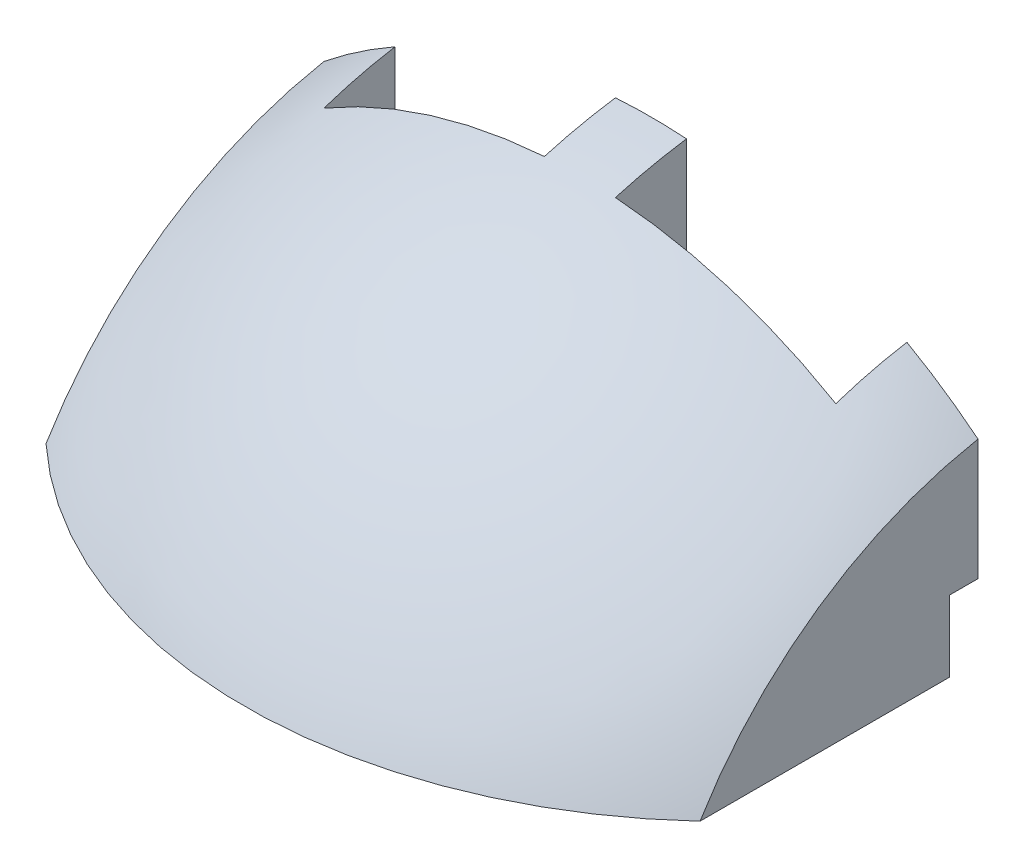
# Autodesk Inventor part: body back for main printing
Saved by Autodesk Inventor 2023 (Build 270158000, 158)
## iProperties
Created: 2022-10-08
Part Number: body back for main printing
Material: ABS プラスチック
Document SubType Name: Modeling
Designer: ellie
Density: 1.06 g/cm^3
Appearance: 積雪
Author: ellie
Autodesk Inventor part; units mm, degrees
sketch "スケッチ1" plane through (0, 0, 0) normal (0, 1, 0) x (-1, 0, 0)
  circle A0 centre (0, 0) radius 37
  line L0 (0, 0) -> (0, -37)
  line L1 (0, 0) -> (0, 37)
  dimension "d0" = 74
  constraints: 4 end point, 2 point on circle, 2 vertical, 1 centre point, 1 coincident
  measures "d0" diameter of A0
revolve "回転1" add sketch "スケッチ1" angle 180 about axis through (0, 0, 0) along (0, 0, 1) picked at (-2.7444, -24.3574) contours L1 L0 A0
sketch "スケッチ5" plane through (0, 0, 0) normal (0, -1, 0) x (1, 0, 0)
  line L0 (-20, -25) -> (20, -25)
  line L1 (20, -25) -> (20, -15)
  line L2 (20, -15) -> (-20, -15)
  line L3 (-20, -15) -> (-20, -25)
  line L4 (-20, -17) -> (-20, -15)
  line L5 (0, 27.75) -> (-17, 27.75)
  line L6 (-17, 27.75) -> (-17, 25.75)
  line L7 (-17, 25.75) -> (0, 25.75)
  line L8 (0, 25.75) -> (0, 27.75)
  line L9 (0, 22.75) -> (-20, 22.75)
  line L10 (-20, 22.75) -> (-20, 21.75)
  line L11 (-20, 21.75) -> (0, 21.75)
  line L12 (0, 21.75) -> (0, 22.75)
  line L13 (0, 15.75) -> (-21, 15.75)
  line L14 (-21, 15.75) -> (-21, 13.75)
  line L15 (-21, 13.75) -> (0, 13.75)
  line L16 (0, 13.75) -> (0, 15.75)
  line L17 (0, 7.75) -> (-23, 7.75)
  line L18 (-23, 7.75) -> (-23, 5.25)
  line L19 (-23, 5.25) -> (0, 5.25)
  line L20 (0, 5.25) -> (0, 7.75)
  circle A0 centre (0, 0) radius 37 projected
  circle A1 centre (0, 0) radius 37 projected
  line L21 (0, 37) -> (0, -37)
  line L22 (37, 0) -> (-37, 0)
  line L23 (-32.5, 5.25) -> (-23, 5.25)
  line L24 (-23, 5.25) -> (-23, -5.25)
  line L25 (-23, -5.25) -> (-32.5, -5.25)
  line L26 (-32.5, -5.25) -> (-32.5, 5.25)
  line L27 (-23, -8.0262) -> (-23, 5.25)
  line L28 (-27, 25.2982) -> (-27, -25.2982)
  line L29 (-15.5, 27.75) -> (-12, 27.75)
  line L30 (-12, 27.75) -> (-12, 35)
  line L31 (-12, 35) -> (-15.5, 35)
  line L32 (-15.5, 35) -> (-15.5, 27.75)
  line L33 (-15.5, 25.75) -> (0, 25.75)
  line L34 (0, 25.75) -> (0, 22.75)
  line L35 (0, 22.75) -> (-15.5, 22.75)
  line L36 (-15.5, 22.75) -> (-15.5, 25.75)
  line L37 (-19, 15.75) -> (0, 15.75)
  line L38 (0, 15.75) -> (0, 21.75)
  line L39 (0, 21.75) -> (-19, 21.75)
  line L40 (-19, 21.75) -> (-19, 15.75)
  line L41 (-19, 13.75) -> (0, 13.75)
  line L42 (0, 13.75) -> (0, 7.75)
  line L43 (0, 7.75) -> (-19, 7.75)
  line L44 (-19, 7.75) -> (-19, 13.75)
  line L45 (-23, 0) -> (-40.624, 0)
  line L46 (-23, 0) -> (-8.7712, 0)
  line L47 (-9.875, 5.25) -> (-23, 5.25)
  line L48 (-23, 5.25) -> (-23, -5.25)
  line L49 (-23, -5.25) -> (-9.875, -5.25)
  line L50 (-9.875, 5.25) -> (-23, -5.25) construction
  line L51 (-23, 5.25) -> (-9.875, -5.25) construction
  line L52 (-23, 7.25) -> (-33.5, 7.25)
  line L53 (-33.5, 7.25) -> (-33.5, -7.25)
  line L54 (-33.5, -7.25) -> (-23, -7.25)
  line L55 (-23, -7.25) -> (-23, 7.25)
  line L56 (-23, 7.25) -> (-33.5, -7.25) construction
  line L57 (-33.5, 7.25) -> (-23, -7.25) construction
  line L58 (-6.125, 5.25) -> (0, 5.25)
  line L59 (0, 5.25) -> (0, -5.25)
  line L60 (0, -5.25) -> (-6.125, -5.25)
  line L61 (-6.125, 5.25) -> (0, -5.25) construction
  line L62 (0, 5.25) -> (-6.125, -5.25) construction
  line L63 (-23, 5.25) -> (-27, 5.25)
  line L64 (-23, -5.25) -> (-27, -5.25)
  line L65 (-23, 7.25) -> (-27, 7.25)
  line L66 (-23, -7.25) -> (-27, -7.25)
  line L67 (26.3249, -26) -> (-26.3249, -26)
  line L68 (-6.125, 5.25) -> (-6.8, 5.25)
  line L69 (-6.2297, -5.25) -> (-6.125, -5.25)
  line L70 (-6.125, -5.25) -> (-6.125, 5.25)
  line L71 (-3, 7.75) -> (0, 7.75)
  line L72 (0, 22.75) -> (-4, 22.75)
  line L73 (-4, 21.75) -> (0, 21.75)
  line L74 (0, 21.75) -> (0, 22.75)
  line L75 (-6, 7.75) -> (-1, 7.75)
  line L76 (0, 5.25) -> (-6, 5.25)
  point P0 (0, -25)
  point P1 (0, -15)
  point P2 (0, 26.75)
  point P3 (0, 22.25)
  point P4 (0, 14.75)
  point P5 (0, 6.5)
  point P6 (-20, -20)
  point P7 (-27, -0.5262)
  point P8 (-27, -5.25)
  point P9 (-15.5, 24.25)
  point P10 (-15.5, 33.5969)
  point P11 (0, 27.75)
  point P12 (0, 37)
  point P13 (0, 25.75)
  point P14 (0, 13.75)
  point P15 (0, 15.75)
  point P16 (-27, 0)
  point P17 (-32.5, 0)
  point P18 (-23, 0)
  point P19 (-16.4375, 0)
  point P20 (-28.25, 0)
  point P21 (-3.0625, 0)
  point P22 (-27, 0.5)
  point P23 (-28, 0.4738)
  point P24 (-28, -11.5262)
  point P25 (-27, -11.5)
  point P26 (-23, -5.25)
  point P27 (-23, 5.25)
  point P28 (-23, -5.25)
  point P29 (0, 0)
  point P30 (-8, 6)
  point P31 (-26.3249, -26)
  point P32 (-8, -6)
  point P33 (0, 21.75)
  point P34 (0, 22.75)
  point P35 (-27, -7.25)
  point P36 (-27, 7.25)
  point P37 (-19, 10.75)
  dimension "d12" = 40
  dimension "d13" = 10
  dimension "d23" = 17
  dimension "d24" = 2
  dimension "d27" = 20
  dimension "d28" = 1
  dimension "d30" = 21
  dimension "d31" = 2
  dimension "d33" = 2.5
  dimension "d88" = 0
  dimension "d89" = 0
  dimension "d90" = 12
  dimension "d92" = 20
  dimension "d97" = 9.5
  dimension "d98" = 10.5
  dimension "d113" = 27
  dimension "d122" = 15.5
  dimension "d124" = 3
  dimension "d125" = 15.5
  dimension "d126" = 6
  dimension "d127" = 6
  dimension "d147" = 10.5
  dimension "d161" = 14.5
  dimension "d162" = 10.5
  dimension "d164" = 10.5
  dimension "d170" = 26
  dimension "d207" = 0
  dimension "d283" = 2
  dimension "d284" = 2
  dimension "d297" = 23
  constraints: 152 end point, 28 parallel, 20 horizontal, 16 midpoint, 16 perpendicular, 16 point on line, 10 collinear, 1 vertical, 20 other
  measures "d12" distance of L2.end L1.end
  measures "d13" distance of L1.end L0.end
  measures "d23" distance of L7.end L6.end
  measures "d24" distance of L6.end L5.end
  measures "d27" distance of L11.end L10.end
  measures "d28" distance of L10.end L9.end
  measures "d30" distance of L15.end L14.end
  measures "d31" distance of L14.end L13.end
  measures "d33" distance of L18.end L17.end
  measures "d89" distance from line of point (0, 0) L22
  measures "d90" distance from line of L0 point (0, -37)
  measures "d92" distance of the line from the sketch origin of L3
  measures "d97" distance of L24.end L25.end
  measures "d98" distance of L23.end L24.end
  measures "d113" distance of the line from the sketch origin of L28
  measures "d122" distance of the line from the sketch origin of L32
  measures "d124" distance of L33.end L34.end
  measures "d126" distance of L38.end L37.end
  measures "d127" distance of L41.end L42.end
  measures "d147" distance of L48.end L47.end
  measures "d161" distance between parallel lines of L54 L52
  measures "d162" distance between parallel lines of L48 L53
  measures "d164" distance between parallel lines of L60 L58
  measures "d170" distance between parallel lines of L67 L22
  measures "d207" distance between parallel lines of L47 L19
  measures "d283" distance from line of L14 point (-19, 10.75)
  measures "d284" distance between parallel lines of L14 L40
  measures "d297" distance between parallel lines of L27 L59
extrude "GNSボード" cut sketch "スケッチ5" against normal blind 16 contours L8 L7 L6 L5
extrude "GNSボード止めるよう" cut sketch "スケッチ5" against normal blind 15 contours L21 L5 L30 A0 | L30 L5 L32 A0 | L21 L9 L36 L7
extrude "アルミ板１" cut sketch "スケッチ5" against normal blind 20 contours L12 L11 L10 L9
extrude "メイン基板" cut sketch "スケッチ5" against normal blind 21 contours L15 L14 L13 L16
extrude "メイン止めるよう" cut sketch "スケッチ5" against normal blind 14.5 contours L17 L44 L15 L21 | L13 L40 L11 L21
extrude "アルミ板２" cut sketch "スケッチ5" against normal blind 20 contours L19 L18 L17 L20
extrude "電池ボックス入れ" cut sketch "スケッチ5" against normal blind 13 contours L3 L2 L21 L0 | L21 L2 L1 L0
extrude "side ut" cut sketch "スケッチ5" against normal blind 100 contours A0 L22 L53 L54 L28 | A0 L28 L52 L53 L22 | L54 L53 L22 L26 L25 L28 | L53 L52 L28 L23 L26 L22 | L25 L26 L22 L28 | L26 L23 L28 L22
extrude "motor case" add sketch "スケッチ5" against normal blind 7 contours L54 L53 L22 L26 L25 L28 | L28 L25 L27 L54 | L53 L52 L28 L23 L26 L22 | L28 L22 L24 L25 | L25 L26 L22 L28 | L22 L28 L23 L24 | L52 L18 L23 L28 | L26 L23 L28 L22
extrude "bottom cut" cut sketch "スケッチ5" against normal blind 90 contours L67 A0 L21 | L21 A0 L67
extrude "motor" [suppressed]
extrude "motor block" [suppressed]
sketch "スケッチ27" plane through (-33.5, 0, -7.25) normal (-1, 0, 0) x (0, 0, 1)
  line L0 (14.5, 0) -> (0, 0) projected
  circle A0 centre (7.25, 0) radius 3
  point P0 (7.25, 0)
  dimension "d198" = 6
  constraints: 1 centre point, 1 midpoint
  measures "d198" diameter of A0
extrude "押し出し36" cut sketch "スケッチ27" against normal blind 27
mirror "ミラー13" about plane through (0, 0, 0) normal (1, 0, 0) of "メイン止めるよう", "メイン基板", "アルミ板１", "GNSボード止めるよう", "GNSボード", "アルミ板２", "motor case", "押し出し36", "電池ボックス入れ", "side ut"
ref_plane "作業平面5" through (-17, 17.5, 25.75) normal (0, -1, 0) x (1, 0, 0)
ref_plane "作業平面6" through (20, 13, -15) normal (0, 0, -1) x (1, 0, 0)
sketch "スケッチ38" plane through (20, 13, -15) normal (0, 0, -1) x (1, 0, 0)
  line L0 (-40, 13) -> (0, 13) projected
  line L1 (-40, 13) -> (-40, 0) projected
  line L2 (-40, 0) -> (0, 0) projected
  line L3 (0, 13) -> (0, 0) projected
  line L4 (-38, 6) -> (-28, 6)
  line L5 (-28, 6) -> (-28, -3)
  line L6 (-28, -3) -> (-38, -3)
  line L7 (-38, -3) -> (-38, 6)
  point P0 (-20, 13)
  dimension "d235" = 3
  dimension "d236" = 9
  dimension "d237" = 10
  dimension "d238" = 2
  constraints: 8 end point, 2 parallel, 1 horizontal, 1 perpendicular
  measures "d235" distance between parallel lines of L6 L2
  measures "d236" distance between parallel lines of L6 L4
  measures "d237" distance between parallel lines of L7 L5
  measures "d238" distance between parallel lines of L1 L7
extrude "押し出し44" cut sketch "スケッチ38" against normal blind 18 contours L7 L4 L5 L2 | L2 L5 L6 L7
ref_plane "作業平面7" through (27, 35, 7.25) normal (0, -1, 0) x (1, 0, 0)
sketch "スケッチ41" plane through (-17, 0, 25.75) normal (0, -1, 0) x (1, 0, 0)
  line L0 (-16.5, -22.75) -> (10.5, -22.75) projected
  line L1 (-6, -20.5) -> (-6, -18) projected
  line L2 (-6, -18) -> (-2, -18) projected
  line L3 (-2, -18) -> (-2, -12) projected
  line L4 (-2, -12) -> (-4, -12) projected
  line L5 (-4, -12) -> (-4, -10) projected
  line L6 (-4, -10) -> (-2, -10) projected
  line L7 (-2, -10) -> (-2, -4) projected
  line L8 (-2, -4) -> (-3, -4) projected
  line L9 (-3, -4) -> (-3, -3) projected
  line L10 (-3, -3) -> (1.5, -3) projected
  line L11 (1.5, -3) -> (1.5, 0) projected
  line L12 (1.5, 0) -> (0, 0) projected
  line L13 (0, 0) -> (0, 2) projected
  line L14 (0, 2) -> (1.5, 2) projected
  line L15 (1.5, 2) -> (1.5, 7.8469) projected
  arc A0 (1.5, 7.8469) -> (-10, -0.4518) centre (17, -25.75) ccw projected
  line L16 (-10, -0.4518) -> (-10, -18.5) projected
  line L17 (-10, -18.5) -> (-16.5, -18.5) projected
  line L18 (-16.5, -18.5) -> (-16.5, -22.75) projected
  line L19 (-2, -18) -> (-2, -12) projected
  line L20 (-4, -10) -> (-4, -12) projected
  line L21 (0, 2) -> (0, 0) projected
  circle A1 centre (-4, 0) radius 2
  line L22 (50.5, -28.75) -> (23.5, -28.75) projected
  line L23 (23.5, -28.75) -> (23.5, -22.75) projected
  line L24 (23.5, -22.75) -> (50.5, -22.75) projected
  line L25 (50.5, -18.5) -> (50.5, -22.75) projected
  line L26 (44, -18.5) -> (50.5, -18.5) projected
  line L27 (44, -18.5) -> (44, -0.4518) projected
  arc A2 (44, -0.4518) -> (32.5, 7.8469) centre (17, -25.75) ccw projected
  line L28 (32.5, 7.8469) -> (32.5, 2) projected
  line L29 (32.5, 2) -> (34, 2) projected
  line L30 (34, 2) -> (34, 0) projected
  line L31 (34, 0) -> (32.5, 0) projected
  line L32 (32.5, 0) -> (32.5, -3) projected
  line L33 (32.5, -3) -> (37, -3) projected
  line L34 (37, -3) -> (37, -4) projected
  line L35 (37, -4) -> (36, -4) projected
  line L36 (36, -4) -> (36, -10) projected
  line L37 (36, -10) -> (38, -10) projected
  line L38 (38, -10) -> (38, -12) projected
  line L39 (38, -12) -> (36, -12) projected
  line L40 (36, -12) -> (36, -18) projected
  line L41 (36, -18) -> (40, -18) projected
  line L42 (40, -18) -> (40, -20.5) projected
  line L43 (40, -20.5) -> (-6, -20.5) projected
  line L44 (10.5, -22.75) -> (10.5, -28.75) projected
  line L45 (10.5, -28.75) -> (-16.5, -28.75) projected
  line L46 (-16.5, -28.75) -> (-16.5, -33) projected
  line L47 (-16.5, -33) -> (-10, -33) projected
  line L48 (-10, -33) -> (-10, -51.0482) projected
  arc A3 (-10, -51.0482) -> (-9.3249, -51.75) centre (17, -25.75) ccw projected
  line L49 (-9.3249, -51.75) -> (43.3249, -51.75) projected
  arc A4 (43.3249, -51.75) -> (44, -51.0482) centre (17, -25.75) ccw projected
  line L50 (44, -51.0482) -> (44, -33) projected
  line L51 (50.5, -33) -> (44, -33) projected
  line L52 (50.5, -28.75) -> (50.5, -33) projected
  dimension "d252" = 4
  dimension "d253" = 4
  dimension "d254" = 3
  constraints: 1 centre point
  measures "d252" diameter of A1
  measures "d253" distance from line of A1.centre L13
  measures "d254" distance from line of A1.centre L10
extrude "押し出し46" cut sketch "スケッチ41" against normal blind 10 contours A1
mirror "ミラー15" about plane through (0, 0, 0) normal (1, 0, 0) of "押し出し46"
sketch "スケッチ42" plane through (-33.5, 0, -7.25) normal (0, -1, 0) x (1, 0, 0)
  circle A0 centre (10, -8) radius 2
  line L0 (13.5, -17.75) -> (13.5, -7.75) projected
  line L1 (10, 2) -> (1, 2) projected
  point P0 (33.5, 7.25)
  dimension "d257" = 3.5
  dimension "d258" = 4
  dimension "d259" = 10
  constraints: 1 centre point
  measures "d257" distance from line of A0.centre L0
  measures "d258" diameter of A0
  measures "d259" distance from line of A0.centre L1
extrude "押し出し47" cut sketch "スケッチ42" against normal blind 10
mirror "ミラー16" about plane through (0, 0, 0) normal (1, 0, 0) of "押し出し47"
ref_plane "作業平面8" through (-17, 15, 25.75) normal (0, -1, 0) x (1, 0, 0)
sketch "スケッチ45" plane through (-17, 15, 25.75) normal (0, -1, 0) x (1, 0, 0)
  circle A0 centre (-4, 0) radius 2 projected
  line L0 (-16.5, -22.75) -> (10.5, -22.75) projected
  line L1 (-6, -20.5) -> (-6, -18) projected
  line L2 (-6, -18) -> (-2, -18) projected
  line L3 (-2, -18) -> (-2, -12) projected
  line L4 (-2, -12) -> (-4, -12) projected
  line L5 (-4, -12) -> (-4, -10) projected
  line L6 (-4, -10) -> (-2, -10) projected
  line L7 (-2, -10) -> (-2, -4) projected
  line L8 (-2, -4) -> (-3, -4) projected
  line L9 (-3, -4) -> (-3, -3) projected
  line L10 (-3, -3) -> (1.5, -3) projected
  line L11 (1.5, -3) -> (1.5, 0) projected
  line L12 (1.5, 0) -> (0, 0) projected
  line L13 (0, 0) -> (0, 2) projected
  line L14 (0, 2) -> (1.5, 2) projected
  line L15 (1.5, 2) -> (1.5, 7.8469) projected
  arc A1 (1.5, 7.8469) -> (-10, -0.4518) centre (17, -25.75) ccw projected
  line L16 (-10, -0.4518) -> (-10, -18.5) projected
  line L17 (-10, -18.5) -> (-16.5, -18.5) projected
  line L18 (-16.5, -18.5) -> (-16.5, -22.75) projected
  arc A2 (32.5, 4.3124) -> (1.5, 4.3124) centre (17, -25.75) ccw projected
  line L19 (1.5, 2) -> (1.5, 4.3124) projected
  line L20 (32.5, 2) -> (1.5, 2) projected
  line L21 (32.5, 2) -> (32.5, 4.3124) projected
  circle A3 centre (38, 0) radius 2 projected
  circle A4 centre (38, 0) radius 2 projected
  line L22 (23.5, -22.75) -> (50.5, -22.75) projected
  line L23 (50.5, -18.5) -> (50.5, -22.75) projected
  line L24 (44, -18.5) -> (50.5, -18.5) projected
  line L25 (44, -18.5) -> (44, -0.4518) projected
  arc A5 (44, -0.4518) -> (32.5, 7.8469) centre (17, -25.75) ccw projected
  line L26 (32.5, 7.8469) -> (32.5, 2) projected
  line L27 (32.5, 2) -> (34, 2) projected
  line L28 (34, 2) -> (34, 0) projected
  line L29 (34, 0) -> (32.5, 0) projected
  line L30 (32.5, 0) -> (32.5, -3) projected
  line L31 (32.5, -3) -> (37, -3) projected
  line L32 (37, -3) -> (37, -4) projected
  line L33 (37, -4) -> (36, -4) projected
  line L34 (36, -4) -> (36, -10) projected
  line L35 (36, -10) -> (38, -10) projected
  line L36 (38, -10) -> (38, -12) projected
  line L37 (38, -12) -> (36, -12) projected
  line L38 (36, -12) -> (36, -18) projected
  line L39 (36, -18) -> (40, -18) projected
  line L40 (40, -18) -> (40, -20.5) projected
  circle A6 centre (-4, 0) radius 2 projected
  line L41 (1.5, 0) -> (32.5, 0) projected
  line L42 (32.5, -3) -> (1.5, -3) projected
  line L43 (32.5, -3) -> (32.5, 0) projected
  line L44 (1.5, 0) -> (32.5, 0) projected
  line L45 (1.5, -3) -> (1.5, 0) projected
  line L46 (34, 0) -> (0, 0) projected
  line L47 (34, 0) -> (34, 2) projected
  line L48 (34, 2) -> (0, 2) projected
  line L49 (0, 0) -> (0, 2) projected
  line L50 (36, -10) -> (-2, -10) projected
  line L51 (36, -10) -> (36, -4) projected
  line L52 (-2, -4) -> (36, -4) projected
  line L53 (-2, -10) -> (-2, -4) projected
  line L54 (38, -12) -> (-4, -12) projected
  line L55 (38, -12) -> (38, -10) projected
  line L56 (38, -10) -> (-4, -10) projected
  line L57 (-4, -12) -> (-4, -10) projected
  line L58 (36, -18) -> (-2, -18) projected
  line L59 (36, -18) -> (36, -12) projected
  line L60 (-2, -12) -> (36, -12) projected
  line L61 (-2, -18) -> (-2, -12) projected
  line L62 (40, -20.5) -> (-6, -20.5) projected
  line L63 (40, -20.5) -> (40, -18) projected
  line L64 (40, -18) -> (-6, -18) projected
  line L65 (-6, -20.5) -> (-6, -18) projected
  circle A7 centre (40.5, -41) radius 2 projected
  circle A8 centre (-6.5, -41) radius 2 projected
  line L66 (50.5, -28.75) -> (23.5, -28.75) projected
  line L67 (40, -20.5) -> (-6, -20.5) projected
  line L68 (10.5, -28.75) -> (-16.5, -28.75) projected
  line L69 (-6, -20.5) -> (-6, -18) projected
  line L70 (-16.5, -28.75) -> (-16.5, -33) projected
  line L71 (-16.5, -33) -> (-10, -33) projected
  line L72 (-10, -33) -> (-10, -51.0482) projected
  arc A9 (-10, -51.0482) -> (-9.3249, -51.75) centre (17, -25.75) ccw projected
  line L73 (-9.3249, -51.75) -> (43.3249, -51.75) projected
  arc A10 (43.3249, -51.75) -> (44, -51.0482) centre (17, -25.75) ccw projected
  line L74 (44, -51.0482) -> (44, -33) projected
  line L75 (50.5, -33) -> (44, -33) projected
  line L76 (50.5, -28.75) -> (50.5, -33) projected
  line L77 (40, -18) -> (40, -20.5) projected
  line L78 (-3, -40.75) -> (37, -40.75) projected
  line L79 (37, -40.75) -> (37, -50.75) projected
  line L80 (37, -50.75) -> (-3, -50.75) projected
  line L81 (-3, -50.75) -> (-3, -40.75) projected
  line L82 (-6, -18) -> (40, -18)
  line L83 (40, -18) -> (40, 8.0731)
  line L84 (40, 8.0731) -> (-6, 8.0731)
  line L85 (-6, 8.0731) -> (-6, -18)
  arc A11 (32.5, 4.3124) -> (1.5, 4.3124) centre (17, -25.75) ccw projected
  line L86 (32.5, 4.3124) -> (32.5, 7.8469) projected
  arc A12 (44, -0.4518) -> (32.5, 7.8469) centre (17, -25.75) ccw projected
  line L87 (44, -0.4518) -> (44, -51.0482) projected
  arc A13 (43.3249, -51.75) -> (44, -51.0482) centre (17, -25.75) ccw projected
  line L88 (43.3249, -51.75) -> (-9.3249, -51.75) projected
  arc A14 (-10, -51.0482) -> (-9.3249, -51.75) centre (17, -25.75) ccw projected
  line L89 (-10, -51.0482) -> (-10, -0.4518) projected
  arc A15 (1.5, 7.8469) -> (-10, -0.4518) centre (17, -25.75) ccw projected
  line L90 (1.5, 7.8469) -> (1.5, 4.3124) projected
  line L91 (9, -32) -> (9, -20) projected
  line L92 (-6, -20) -> (9, -20) projected
  line L93 (-6, -21) -> (-6, -20) projected
  line L94 (-15, -21) -> (-6, -21) projected
  line L95 (-15, -31) -> (-15, -21) projected
  line L96 (-6, -31) -> (-15, -31) projected
  line L97 (-6, -32) -> (-6, -31) projected
  line L98 (9, -32) -> (-6, -32) projected
  line L99 (50.5, -28.75) -> (23.5, -28.75) projected
  line L100 (50.5, -22.75) -> (50.5, -28.75) projected
  line L101 (23.5, -22.75) -> (50.5, -22.75) projected
  line L102 (-16.5, -22.75) -> (10.5, -22.75) projected
  line L103 (-16.5, -28.75) -> (-16.5, -22.75) projected
  line L104 (10.5, -28.75) -> (-16.5, -28.75) projected
  line L105 (10.5, -28.75) -> (10.5, -22.75) projected
  line L106 (23.5, -28.75) -> (23.5, -22.75) projected
  line L107 (50.5, -28.75) -> (23.5, -28.75) projected
  line L108 (23.5, -28.75) -> (23.5, -22.75) projected
  line L109 (40, -20.5) -> (-6, -20.5) projected
  line L110 (-6, -20.5) -> (-6, -18) projected
  line L111 (-6, -18) -> (-2, -18) projected
  line L112 (-2, -18) -> (-2, -12) projected
  line L113 (-2, -12) -> (-4, -12) projected
  line L114 (-4, -12) -> (-4, -10) projected
  line L115 (-4, -10) -> (-2, -10) projected
  line L116 (-2, -10) -> (-2, -4) projected
  line L117 (-2, -4) -> (-3, -4) projected
  line L118 (-3, -4) -> (-3, -3) projected
  line L119 (-3, -3) -> (1.5, -3) projected
  line L120 (1.5, -3) -> (1.5, 0) projected
  line L121 (1.5, 0) -> (0, 0) projected
  line L122 (0, 0) -> (0, 2) projected
  line L123 (0, 2) -> (1.5, 2) projected
  line L124 (1.5, 2) -> (1.5, 7.8469) projected
  arc A16 (1.5, 7.8469) -> (-10, -0.4518) centre (17, -25.75) ccw projected
  line L125 (-10, -0.4518) -> (-10, -18.5) projected
  line L126 (-10, -18.5) -> (-16.5, -18.5) projected
  line L127 (-16.5, -18.5) -> (-16.5, -22.75) projected
  line L128 (-16.5, -22.75) -> (10.5, -22.75) projected
  line L129 (10.5, -22.75) -> (10.5, -28.75) projected
  line L130 (10.5, -28.75) -> (-16.5, -28.75) projected
  line L131 (-16.5, -28.75) -> (-16.5, -33) projected
  line L132 (-16.5, -33) -> (-10, -33) projected
  line L133 (-10, -33) -> (-10, -51.0482) projected
  arc A17 (-10, -51.0482) -> (-9.3249, -51.75) centre (17, -25.75) ccw projected
  line L134 (-9.3249, -51.75) -> (43.3249, -51.75) projected
  arc A18 (43.3249, -51.75) -> (44, -51.0482) centre (17, -25.75) ccw projected
  line L135 (44, -51.0482) -> (44, -33) projected
  line L136 (50.5, -33) -> (44, -33) projected
  line L137 (50.5, -28.75) -> (50.5, -33) projected
  line L138 (50.5, -28.75) -> (23.5, -28.75) projected
  line L139 (23.5, -28.75) -> (23.5, -22.75) projected
  line L140 (23.5, -22.75) -> (50.5, -22.75) projected
  line L141 (50.5, -18.5) -> (50.5, -22.75) projected
  line L142 (44, -18.5) -> (50.5, -18.5) projected
  line L143 (44, -18.5) -> (44, -0.4518) projected
  arc A19 (44, -0.4518) -> (32.5, 7.8469) centre (17, -25.75) ccw projected
  line L144 (32.5, 7.8469) -> (32.5, 2) projected
  line L145 (32.5, 2) -> (34, 2) projected
  line L146 (34, 2) -> (34, 0) projected
  line L147 (34, 0) -> (32.5, 0) projected
  line L148 (32.5, 0) -> (32.5, -3) projected
  line L149 (32.5, -3) -> (37, -3) projected
  line L150 (37, -3) -> (37, -4) projected
  line L151 (37, -4) -> (36, -4) projected
  line L152 (36, -4) -> (36, -10) projected
  line L153 (36, -10) -> (38, -10) projected
  line L154 (38, -10) -> (38, -12) projected
  line L155 (38, -12) -> (36, -12) projected
  line L156 (36, -12) -> (36, -18) projected
  line L157 (36, -18) -> (40, -18) projected
  line L158 (40, -18) -> (40, -20.5) projected
  line L159 (40, -20.5) -> (-6, -20.5) projected
  line L160 (10.5, -22.75) -> (10.5, -28.75) projected
  line L161 (10.5, -28.75) -> (-16.5, -28.75) projected
  line L162 (-16.5, -28.75) -> (-16.5, -33) projected
  line L163 (-16.5, -33) -> (-10, -33) projected
  line L164 (-10, -33) -> (-10, -51.0482) projected
  arc A20 (-10, -51.0482) -> (-9.3249, -51.75) centre (17, -25.75) ccw projected
  line L165 (-9.3249, -51.75) -> (43.3249, -51.75) projected
  arc A21 (43.3249, -51.75) -> (44, -51.0482) centre (17, -25.75) ccw projected
  line L166 (44, -51.0482) -> (44, -33) projected
  line L167 (50.5, -33) -> (44, -33) projected
  line L168 (50.5, -28.75) -> (50.5, -33) projected
  line L169 (23.5, -28.75) -> (23.5, -22.75) projected
  line L170 (23.5, -22.75) -> (50.5, -22.75) projected
  line L171 (50.5, -18.5) -> (50.5, -22.75) projected
  line L172 (44, -18.5) -> (50.5, -18.5) projected
  line L173 (44, -18.5) -> (44, -0.4518) projected
  arc A22 (44, -0.4518) -> (32.5, 7.8469) centre (17, -25.75) ccw projected
  line L174 (32.5, 7.8469) -> (32.5, 2) projected
  line L175 (32.5, 2) -> (34, 2) projected
  line L176 (34, 2) -> (34, 0) projected
  line L177 (34, 0) -> (32.5, 0) projected
  line L178 (32.5, 0) -> (32.5, -3) projected
  line L179 (32.5, -3) -> (37, -3) projected
  line L180 (37, -3) -> (37, -4) projected
  line L181 (37, -4) -> (36, -4) projected
  line L182 (36, -4) -> (36, -10) projected
  line L183 (36, -10) -> (38, -10) projected
  line L184 (38, -10) -> (38, -12) projected
  line L185 (38, -12) -> (36, -12) projected
  line L186 (36, -12) -> (36, -18) projected
  line L187 (36, -18) -> (40, -18) projected
  line L188 (-6, -18) -> (-2, -18) projected
  line L189 (-2, -18) -> (-2, -12) projected
  line L190 (-2, -12) -> (-4, -12) projected
  line L191 (-4, -12) -> (-4, -10) projected
  line L192 (-4, -10) -> (-2, -10) projected
  line L193 (-2, -10) -> (-2, -4) projected
  line L194 (-2, -4) -> (-3, -4) projected
  line L195 (-3, -4) -> (-3, -3) projected
  line L196 (-3, -3) -> (1.5, -3) projected
  line L197 (1.5, -3) -> (1.5, 0) projected
  line L198 (1.5, 0) -> (0, 0) projected
  line L199 (0, 0) -> (0, 2) projected
  line L200 (0, 2) -> (1.5, 2) projected
  line L201 (1.5, 2) -> (1.5, 7.8469) projected
  arc A23 (1.5, 7.8469) -> (-10, -0.4518) centre (17, -25.75) ccw projected
  line L202 (-10, -0.4518) -> (-10, -18.5) projected
  line L203 (-10, -18.5) -> (-16.5, -18.5) projected
  line L204 (-16.5, -18.5) -> (-16.5, -22.75) projected
  line L205 (-16.5, -22.75) -> (10.5, -22.75) projected
  line L206 (10.5, -22.75) -> (10.5, -28.75) projected
  point P0 (-10, -33)
  point P1 (44, -33)
  point P2 (44, -18.5)
  point P3 (40, 3.2328)
  point P4 (40, -18)
  point P5 (-6, -20.5)
  point P6 (-6, -18)
  point P7 (-6, 3.2328)
  point P8 (-10, -33)
  point P9 (44, -33)
  point P10 (44, -18.5)
  point P11 (-10, -18.5)
  point P12 (44, -22.75)
  point P13 (-10, -22.75)
  point P14 (-10, -18.5)
  point P15 (44, -28.75)
  point P16 (-10, -28.75)
  point P17 (32.5, 4.3124)
  point P18 (1.5, 4.3124)
  point P19 (1.5, 4.3124)
  point P20 (32.5, 4.3124)
  point P21 (-10, -22.75)
  point P22 (-10, -28.75)
  point P23 (32.5, 4.3124)
  point P24 (1.5, 4.3124)
  point P25 (44, -22.75)
  point P26 (44, -28.75)
  point P27 (-10, -18.5)
  point P28 (50.5, -28.75)
  point P29 (44, -33)
  point P30 (1.5, 4.3124)
  point P31 (32.5, 4.3124)
  point P32 (50.5, -28.75)
  point P33 (44, -28.75)
  point P34 (44, -22.75)
  point P35 (32.5, 4.3124)
  point P36 (1.5, 4.3124)
  point P37 (44, -33)
  point P38 (-10, -22.75)
  point P39 (-10, -28.75)
  point P40 (1.5, 4.3124)
  point P41 (32.5, 4.3124)
  point P42 (-16.5, -28.75)
  point P43 (-16.5, -28.75)
  constraints: 8 end point, 3 collinear, 2 parallel, 1 horizontal, 1 perpendicular, 1 tangent
extrude "side and front cut" cut sketch "スケッチ45" along normal mid plane 100 contours L85 L1 L93 L94 L89 L16 A1 | L89 L94 L95 L0 L18 L17 | L62 L91 L0 L89 L94 L93 | L89 L0 L95 L94 | L62 L40 L83 A5 L25 L87 L22 L106 L66 L74 A10 L73 A9 L72 L89 L96 L97 L98 L91 L68 L105 L0 | L0 L95 L68 L103 | L89 L68 L95 L0 | L0 L91 L68 L89 | L0 L105 L68 L91 | L68 L95 L96 L89 L71 L70 | L89 L96 L95 L68 | L68 L91 L98 L97 L96 L89 | L24 L23 L22 L87 | L87 L66 L106 L22 | L22 L100 L66 L87 | L66 L76 L75 L87 | A7 | A8 | L78 L79 L80 L81
sketch "スケッチ46" plane through (-17, 15, 25.75) normal (0, -1, 0) x (1, 0, 0)
  line L0 (-6, 0) -> (-6, -18) projected
  line L1 (-6, -18) -> (-2, -18) projected
  line L2 (-2, -18) -> (-2, -12) projected
  line L3 (-2, -12) -> (-4, -12) projected
  line L4 (-4, -12) -> (-4, -10) projected
  line L5 (-4, -10) -> (-2, -10) projected
  line L6 (-2, -10) -> (-2, -4) projected
  line L7 (-2, -4) -> (-3, -4) projected
  line L8 (-3, -4) -> (-3, -3) projected
  line L9 (-3, -3) -> (1.5, -3) projected
  line L10 (1.5, -3) -> (1.5, 0) projected
  line L11 (1.5, 0) -> (0, 0) projected
  line L12 (0, 0) -> (0, 2) projected
  line L13 (0, 2) -> (1.5, 2) projected
  line L14 (1.5, 2) -> (1.5, 7.8469) projected
  arc A0 (1.5, 7.8469) -> (-6, 3.2328) centre (17, -25.75) ccw projected
  line L15 (-6, 3.2328) -> (-6, 0) projected
  circle A1 centre (-4, 0) radius 2 projected
  circle A2 centre (-4, 0) radius 2 projected
  line L16 (40, -18) -> (40, 0) projected
  circle A3 centre (38, 0) radius 2 projected
  line L17 (40, 0) -> (40, 3.2328) projected
  arc A4 (40, 3.2328) -> (32.5, 7.8469) centre (17, -25.75) ccw projected
  line L18 (32.5, 7.8469) -> (32.5, 2) projected
  line L19 (32.5, 2) -> (34, 2) projected
  line L20 (34, 2) -> (34, 0) projected
  line L21 (34, 0) -> (32.5, 0) projected
  line L22 (32.5, 0) -> (32.5, -3) projected
  line L23 (32.5, -3) -> (37, -3) projected
  line L24 (37, -3) -> (37, -4) projected
  line L25 (37, -4) -> (36, -4) projected
  line L26 (36, -4) -> (36, -10) projected
  line L27 (36, -10) -> (38, -10) projected
  line L28 (38, -10) -> (38, -12) projected
  line L29 (38, -12) -> (36, -12) projected
  line L30 (36, -12) -> (36, -18) projected
  line L31 (36, -18) -> (40, -18) projected
  arc A5 (32.5, 4.3124) -> (1.5, 4.3124) centre (17, -25.75) ccw projected
  line L32 (1.5, 2) -> (1.5, 4.3124) projected
  line L33 (32.5, 2) -> (1.5, 2) projected
  line L34 (32.5, 2) -> (32.5, 4.3124) projected
  line L35 (34, 0) -> (0, 0) projected
  line L36 (34, 0) -> (34, 2) projected
  line L37 (34, 2) -> (0, 2) projected
  line L38 (0, 0) -> (0, 2) projected
  line L39 (32.5, -3) -> (1.5, -3) projected
  line L40 (32.5, -3) -> (32.5, 0) projected
  line L41 (1.5, 0) -> (32.5, 0) projected
  line L42 (1.5, -3) -> (1.5, 0) projected
  line L43 (36, -10) -> (-2, -10) projected
  line L44 (36, -10) -> (36, -4) projected
  line L45 (-2, -4) -> (36, -4) projected
  line L46 (-2, -10) -> (-2, -4) projected
  line L47 (36, -18) -> (-2, -18) projected
  line L48 (36, -18) -> (36, -12) projected
  line L49 (-2, -12) -> (36, -12) projected
  line L50 (-2, -18) -> (-2, -12) projected
  point P0 (1.5, 4.3124)
  point P1 (-2, -18)
  point P2 (36, -18)
  constraints: 3 horizontal alignment
extrude "front cut 2" cut sketch "スケッチ46" along normal blind 100 contours L15 A0 L14 L13 L12 L11 L10 L9 L8 L7 L6 L5 L4 L3 L2 L1 L0 | A1 | L2 L49 L30 L47 | L3 L4 L5 L43 L27 L28 L29 L49 | A3 | L30 L29 L28 L27 L26 L25 L24 L23 L22 L21 L20 L19 L18 A4 L17 L16 L31 | A5 L18 L33 L14 | L33 L19 L20 L21 L35 L11 L12 L13 | L6 L45 L26 L43 | L7 L8 L9 L39 L23 L24 L25 L45 | L35 L22 L39 L10
sketch "スケッチ48" plane through (0, 0, 5.25) normal (0, 0, -1) x (-1, 0, 0)
  line L0 (-23, 20) -> (23, 20) projected
  line L1 (23, 28.5033) -> (23, 20) projected
  arc A0 (23, 28.5033) -> (-23, 28.5033) centre (0, 0) ccw projected
  line L2 (-23, 28.5033) -> (-23, 20) projected
  line L3 (-23, 15) -> (23, 15) projected
  line L4 (-23, 15) -> (-23, 20) projected
  line L5 (23, 15) -> (23, 20) projected
  line L6 (-23, 40) -> (-18, 40)
  line L7 (-18, 40) -> (-18, 15)
  line L8 (-18, 15) -> (-23, 15)
  line L9 (-23, 15) -> (-23, 40)
  line L10 (18, 40) -> (23, 40)
  line L11 (23, 40) -> (23, 15)
  line L12 (23, 15) -> (18, 15)
  line L13 (18, 15) -> (18, 40)
  line L14 (-2.5, 36.6256) -> (2.5, 36.6256)
  line L15 (2.5, 36.6256) -> (2.5, 20)
  line L16 (2.5, 20) -> (-2.5, 20)
  line L17 (-2.5, 20) -> (-2.5, 36.6256)
  line L18 (0, 0) -> (0, 36.6256)
  point P0 (18, 20)
  point P1 (18, 31.8973)
  point P2 (-18, 31.8973)
  point P3 (-18, 20)
  point P4 (2.5, 36.5402)
  point P5 (2.5, 20)
  point P6 (-2.5, 36.5402)
  dimension "d274" = 25
  dimension "d275" = 5
  dimension "d276" = 25
  dimension "d277" = 5
  dimension "d280" = 5
  dimension "d282" = 2.5
  constraints: 26 end point, 6 parallel, 5 collinear, 3 horizontal, 3 perpendicular, 1 midpoint, 1 point on circle, 1 tangent
  measures "d274" distance between parallel lines of L3 L6
  measures "d275" distance between parallel lines of L9 L7
  measures "d276" distance between parallel lines of L3 L10
  measures "d277" distance between parallel lines of L13 L11
  measures "d280" distance between parallel lines of L17 L15
  measures "d282" distance between parallel lines of L17 L18
extrude "lock cut" cut sketch "スケッチ48" against normal blind 3 contours L7 A0 L17 L0 | L15 A0 L13 L0
sketch "スケッチ49" plane through (23, 15, 7.75) normal (0, 0, -1) x (-1, 0, 0)
  line L0 (46, 0) -> (0, 0) projected
  line L1 (46, -15) -> (46, 5) projected
  line L2 (0, 0) -> (46, 0)
  line L3 (46, 0) -> (46, 5)
  line L4 (46, 5) -> (0, 5)
  line L5 (0, 5) -> (0, 0)
  point P0 (23, -15)
  point P1 (38.5, 0)
  point P2 (7.5, 0)
  constraints: 8 end point, 2 parallel, 1 horizontal, 1 perpendicular
extrude "押し出し52" cut sketch "スケッチ49" against normal up to surface (0.5 mm away)
sketch "スケッチ50" plane through (0, 0, 5.25) normal (0, 0, -1) x (-1, 0, 0)
  point P0 (0, 0)
sketch "スケッチ51" plane through (0, 0, 8.25) normal (0, 0, -1) x (-1, 0, 0)
  line L0 (-23, 15) -> (-23, 28.5033) projected
  line L1 (18, 20) -> (23, 20) projected
  line L2 (-23, 15) -> (23, 15)
  line L3 (23, 15) -> (23, 20)
  line L4 (23, 20) -> (-23, 20)
  line L5 (-23, 20) -> (-23, 15)
  arc A0 (18, 31.256) -> (2.5, 35.9818) centre (0, 0) ccw projected
  line L6 (2.5, 20) -> (2.5, 35.9818) projected
  line L7 (-2.5, 35.9818) -> (-2.5, 20) projected
  arc A1 (-2.5, 35.9818) -> (-18, 31.256) centre (0, 0) ccw projected
  line L8 (-18, 20) -> (-18, 31.256) projected
  line L9 (18, 31.256) -> (18, 20) projected
  line L10 (-2.5, 20) -> (-18, 20) projected
  line L11 (18, 20) -> (2.5, 20) projected
  point P0 (2.5, 20)
  point P1 (-2.5, 20)
  constraints: 8 end point, 2 parallel, 1 horizontal, 1 perpendicular
extrude "押し出し53" cut sketch "スケッチ51" against normal blind 2
sketch "スケッチ52" plane through (0, 0, 10.25) normal (0, 0, -1) x (-1, 0, 0)
  line L0 (-23, 20) -> (-18, 20) projected
  line L1 (-23, 20) -> (-18, 20) projected
  line L2 (-2.5, 20) -> (2.5, 20) projected
  line L3 (-2.5, 20) -> (2.5, 20) projected
  point P0 (0, 0)
sketch "スケッチ53" plane through (0, 15, 0) normal (0, -1, 0) x (1, 0, 0)
  line L0 (18, 10.25) -> (18, 5.25) projected
  line L1 (23, 5.25) -> (18, 5.25) projected
  line L2 (23, 10.25) -> (23, 5.25) projected
  line L3 (23, 10.25) -> (18, 10.25) projected
  line L4 (-2.5, 10.25) -> (-2.5, 5.25) projected
  line L5 (2.5, 5.25) -> (-2.5, 5.25) projected
  line L6 (2.5, 5.25) -> (2.5, 10.25) projected
  line L7 (2.5, 10.25) -> (-2.5, 10.25) projected
  line L8 (-18, 5.25) -> (-18, 10.25) projected
  line L9 (-18, 10.25) -> (-23, 10.25) projected
  line L10 (-23, 5.25) -> (-23, 10.25) projected
  line L11 (-18, 5.25) -> (-23, 5.25) projected
  point P0 (0, 0)
extrude "押し出し54" add sketch "スケッチ53" against normal up to surface (5 mm away)
sketch "スケッチ54" plane through (0, 15, 0) normal (0, -1, 0) x (1, 0, 0)
  line L0 (-18, 10.25) -> (-2.5, 10.25) projected
  line L1 (23, 24.7992) -> (23, 5.25) projected
  line L2 (23, 5.25) -> (-23, 5.25)
  line L3 (-23, 5.25) -> (-23, 7.25)
  line L4 (-23, 7.25) -> (23, 7.25)
  line L5 (23, 7.25) -> (23, 5.25)
  line L6 (18, 5.25) -> (23, 5.25) projected
  point P0 (0, 0)
  point P1 (23, 5.25)
  point P2 (23, 7.25)
  dimension "d295" = 2
  dimension "d296" = 46
  constraints: 8 end point, 2 collinear, 2 parallel, 1 horizontal, 1 perpendicular
  measures "d295" distance between parallel lines of L4 L2
  measures "d296" distance of L3.end L4.end
extrude "押し出し55" cut sketch "スケッチ54" against normal blind 5
